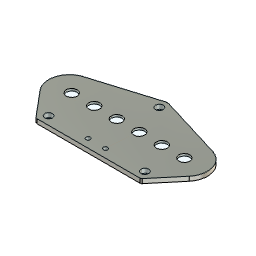
tele_rear_mount v2 (Autodesk Fusion 360 design; units mm, degrees)
Autodesk Fusion 360 part; units mm, degrees
sketch "スケッチ1" plane through (0, 0, 0) normal (0, 0, 1) x (1, 0, 0)
  line L0 (0, 0) -> (72.6, 0)
  line L1 (72.6, 0) -> (72.6, -36.25)
  line L2 (72.6, -36.25) -> (0, -36.25)
  line L3 (0, -36.25) -> (0, 0)
  line L4 (36.3, 0) -> (36.3, -36.25)
  line L5 (0, -18.125) -> (72.6, -18.125)
  line L6 (72.6, -8.625) -> (72.6, -26.625)
  line L7 (58.3, -36.25) -> (14.3, -36.25)
  line L8 (0, -9.125) -> (0, -27.125)
  line L9 (0, -18.125) -> (9.5, -18.125)
  line L10 (0, -9.125) -> (6.4586, -9.125)
  line L11 (0, -27.125) -> (4.6488, -27.125)
  line L12 (6.4586, -9.125) -> (36.3, 0)
  line L13 (14.3, -36.25) -> (12.3, -36.25)
  line L14 (12.3, -36.25) -> (2.2204, -24.2289)
  line L15 (36.3, -18.125) -> (36.3, -32.425)
  line L16 (36.3, -18.125) -> (36.3, -3.825)
  line L17 (66.1414, -9.125) -> (36.3, 0)
  line L18 (60.3, -36.25) -> (70.3796, -24.2289)
  line L19 (58.3, -36.25) -> (60.3, -36.25)
  line L20 (6.4586, -27.125) -> (66.1414, -27.125)
  line L21 (6.4586, -9.125) -> (66.1414, -9.125)
  arc A0 (6.9878, -8.9632) -> (6.4586, -27.125) centre (9.5, -18.125) ccw
  arc A1 (66.1414, -27.125) -> (65.6122, -8.9632) centre (63.1, -18.125) ccw
  circle A2 centre (14.3, -32.425) radius 1.75
  circle A3 centre (36.3, -3.825) radius 1.75
  circle A4 centre (58.3, -32.425) radius 1.75
  circle A5 centre (32.3, -32.425) radius 1
  circle A6 centre (40.3, -32.425) radius 1
  line L22 (36.3, -9.125) -> (36.3, -13.125)
  line L23 (0, -18.125) -> (4, -18.125)
  line L24 (36.3, -13.125) -> (5.4223, -13.125)
  line L25 (36.3, -27.125) -> (36.3, -23.125)
  line L26 (36.3, -23.125) -> (5.4223, -23.125)
  arc A7 (5.4223, -13.125) -> (5.4223, -23.125) centre (13.5, -18.125) ccw
  circle A8 centre (10.55, -18.125) radius 2.5
  circle A9 centre (20.85, -18.125) radius 2.5
  circle A10 centre (31.15, -18.125) radius 2.5
  line L27 (36.3, -13.125) -> (67.1777, -13.125)
  arc A11 (67.1777, -23.125) -> (67.1777, -13.125) centre (59.1, -18.125) ccw
  line L28 (36.3, -23.125) -> (67.1777, -23.125)
  circle A12 centre (62.05, -18.125) radius 2.5
  circle A13 centre (51.75, -18.125) radius 2.5
  circle A14 centre (41.45, -18.125) radius 2.5
  point P0 (36.3, -18.125)
  point P1 (36.3, -3.825)
  point P2 (14.3, -32.425)
  point P3 (58.3, -32.425)
  point P4 (40.3, -32.425)
  point P5 (40.3, -32.425)
  point P6 (32.3, -32.425)
  point P7 (31.15, -18.125)
  point P8 (20.85, -18.125)
  point P9 (10.55, -18.125)
  dimension "d5" = 72.6
  dimension "d6" = 36.25
  dimension "d10" = 44
  dimension "d11" = 9
  dimension "d12" = 18
  dimension "d13" = 9.5
  dimension "d14" = 2
  dimension "d15" = 14.3
  dimension "d16" = 22
  dimension "d17" = 14.3
  dimension "d18" = 3.5
  dimension "d19" = 3.5
  dimension "d20" = 3.5
  dimension "d21" = 4
  dimension "d24" = 2
  dimension "d25" = 2
  dimension "d30" = 4
  dimension "d31" = 4
  dimension "d32" = 9.5
  dimension "d33" = 4
  dimension "d34" = 5.15
  dimension "d35" = 10.3
  dimension "d36" = 10.3
  dimension "d37" = 5
  dimension "d38" = 5
  dimension "d39" = 5
  constraint coincident L0.start L3.end
  constraint horizontal L0
  constraint vertical L1
  constraint horizontal L2
  constraint vertical L3
  constraint midpoint L0 L4.start
  constraint midpoint L2 L4.end
  constraint midpoint L3 L5.start
  constraint midpoint L1 L5.end
  constraint midpoint L5 P0
  constraint vertical L6
  constraint coincident L1 L6.end
  constraint parallel L2 L7
  constraint parallel L3 L8
  constraint perpendicular L8 L9
  constraint perpendicular L3 L10
  constraint perpendicular L8 L11
  constraint parallel L2 L13
  constraint coincident P0 L15.start
  constraint perpendicular L5 L15
  constraint perpendicular L0 L16
  constraint coincident P1 L16.end
  constraint symmetric L4.start L16 L12.end
  constraint symmetric L7.end L16 L7.start
  constraint symmetric L10.end L16 L17.start
  constraint symmetric L13.end L16 L18.start
  constraint symmetric L14.end L16 L18.end
  constraint perpendicular L1 L20
  constraint coincident L12 A0.start
  constraint coincident L17 A1.end
  constraint coincident L14 L11.end
  constraint coincident P2 A2.centre
  constraint coincident P3 A4.centre
  constraint coincident P6 A5.centre
  constraint coincident P5 P4
  constraint midpoint L21 L22.start
  constraint perpendicular L21 L22
  constraint perpendicular L8 L23
  constraint coincident L23.end A7
  constraint perpendicular L4 L24
  constraint midpoint L20 L25.start
  constraint perpendicular L20 L25
  constraint perpendicular L15 L26
  constraint coincident P9 A8.centre
  constraint coincident P8 A9.centre
  constraint coincident P7 A10.centre
  constraint symmetric L4 L22.end L24.start
  constraint symmetric L4 L24.end L27.end
  constraint symmetric L4 L25.end L26.start
  constraint symmetric L4 L26.end A11.start
  constraint symmetric L4 A7 A11
  constraint symmetric L4 A8 A12
  constraint symmetric L4 A9 A13
  constraint symmetric L4 A10 A14
  measures "d5" distance of L0.start L0.end
  measures "d6" distance of L0.start L2.end
  measures "d10" distance of L7.start L7.end
  measures "d11" distance of L5.start L8.start
  measures "d12" distance of L8.start L8.end
  measures "d13" distance of L5.start L9.end
  measures "d14" distance of L7.end L13.end
  measures "d15" distance of P0 L15.end
  measures "d16" distance of L15.end P2
  measures "d17" distance of P0 P1
  measures "d18" diameter of A2
  measures "d19" diameter of A3
  measures "d20" diameter of A4
  measures "d21" distance of L15.end P5
  measures "d24" diameter of A5
  measures "d25" diameter of A6
  measures "d30" distance of L22.start L22.end
  measures "d31" distance of L5.start L23.end
  measures "d32" distance of L23.end A7.centre
  measures "d33" distance of L25.start L25.end
  measures "d34" distance of P0 P7
  measures "d35" distance of P7 P8
  measures "d36" distance of P8 P9
  measures "d37" diameter of A8
  measures "d38" diameter of A9
  measures "d39" diameter of A10
extrude "押し出し1" add sketch "スケッチ1" along normal blind 2 contours L4 L16 L17 L21 A3 | L4 L12 L16 L21 A3 | L4 L5 L9 L16 L21 A0 L22 L23 L24 A7 | L4 L5 L9 L15 L20 A0 L23 L25 L26 A7 | L4 L5 L16 L21 A1 L22 L27 A11 | L4 L5 L9 L16 L24 A7 A8 A9 A10 | L4 L5 L9 L15 L26 A7 A8 A9 A10 | L2 L4 L7 L13 L14 L15 L20 A0 | L4 L5 L15 L20 A1 L25 A11 L28 | L5 L9 A8 | L5 L9 A8 | L4 L5 L16 L27 A11 A12 A13 A14 | L4 L5 L15 A11 L28 A12 A13 A14 | L2 L4 L7 L15 L18 L19 L20 A1 | L5 A12 | L5 A12 | L5 A9 | L5 A9 | L5 A10 | L5 A10 | L5 A14 | L5 A14 | L5 A13 | L5 A13
fillet "フィレット1" radius 1 3 edges at (12.3, -36.25, 1) (60.3, -36.25, 1) (36.3, 0, 1)
sketch "スケッチ2" plane through (0, 0, 2) normal (0, 0, 1) x (-1, 0, 0)
  arc A0 (-36.5924, 0.0894) -> (-36.0076, 0.0894) centre (-36.3, 1.0457) ccw
  line L0 (-36.0076, 0.0894) -> (-6.4586, 9.125)
  arc A1 (-6.4586, 9.125) -> (-2.2204, 24.2289) centre (-9.5, 18.125) ccw
  line L1 (-2.2204, 24.2289) -> (-12.0003, 35.8925)
  arc A2 (-12.0003, 35.8925) -> (-12.7665, 36.25) centre (-12.7665, 35.25) ccw
  line L2 (-12.7665, 36.25) -> (-59.8335, 36.25)
  arc A3 (-59.8335, 36.25) -> (-60.5997, 35.8925) centre (-59.8335, 35.25) ccw
  line L3 (-60.5997, 35.8925) -> (-70.3796, 24.2289)
  arc A4 (-70.3796, 24.2289) -> (-66.1414, 9.125) centre (-63.1, 18.125) ccw
  line L4 (-66.1414, 9.125) -> (-36.5924, 0.0894)
  circle A5 centre (-36.3, 3.825) radius 1.75
  circle A6 centre (-32.3, 32.425) radius 1
  circle A7 centre (-40.3, 32.425) radius 1
  circle A8 centre (-14.3, 32.425) radius 1.75
  circle A9 centre (-58.3, 32.425) radius 1.75
extrude "押し出し2" cut sketch "スケッチ1" along normal blind 1 contours L4 L5 L9 L16 L24 A7 A8 A9 A10 | L4 L5 L9 L15 L26 A7 A8 A9 A10 | L4 L5 L16 L27 A11 A12 A13 A14 | L4 L5 L15 A11 L28 A12 A13 A14
extrude "押し出し3" cut sketch "スケッチ1" along normal blind 2 contours L5 L9 A8 | L5 L9 A8 | L5 A12 | L5 A12 | L5 A9 | L5 A9 | L5 A10 | L5 A10 | L5 A14 | L5 A14 | L5 A13 | L5 A13
fillet "フィレット2" radius 5 4 edges at (5.4223, -13.125, 0.5) (5.4223, -23.125, 0.5) (67.1777, -13.125, 0.5) (67.1777, -23.125, 0.5)
